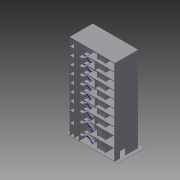
# Autodesk Inventor part: NRCC_Smoke_Tower
Saved by Autodesk Inventor 2013 SP2 (Build 170200200, 200)
## iProperties
Created: 2015-09-15
Part Number: NRCC_Smoke_Tower
Material: Generic
Document SubType Name: Modeling
Designer: mcgratta
Density: 1 g/cm^3
Author: mcgratta
Autodesk Inventor part; units mm, degrees
(part 1 of 2)
sketch "Sketch1" plane through (0, 0, 0) normal (0, 1, 0) x (-1, 0, 0)
  line L0 (-1000, -1000) -> (-1200, -1000)
  line L1 (-1200, -1000) -> (-1200, -10300)
  line L2 (-1200, -10300) -> (-1000, -10300)
  line L3 (-1000, -10300) -> (-1000, -1000)
  line L4 (-1200, -1000) -> (-15700, -1000)
  line L5 (-15700, -1000) -> (-15700, -1200)
  line L6 (-15700, -1200) -> (-1200, -1200)
  line L7 (-1200, -1200) -> (-1200, -1000)
  line L8 (-15700, -1000) -> (-15900, -1000)
  line L9 (-15900, -1000) -> (-15900, -10300)
  line L10 (-15900, -10300) -> (-15700, -10300)
  line L11 (-15700, -10300) -> (-15700, -1000)
  line L12 (-15700, -10300) -> (-15700, -10100)
  line L13 (-1200, -10100) -> (-1200, -10300)
  line L14 (-2400, -2400) -> (-2600, -2400)
  line L15 (-2600, -2400) -> (-2600, -8900)
  line L16 (-2600, -8900) -> (-2400, -8900)
  line L17 (-2400, -8900) -> (-2400, -2400)
  line L18 (-2600, -2400) -> (-11700, -2400)
  line L19 (-11700, -2400) -> (-11700, -2600)
  line L20 (-11700, -2600) -> (-2600, -2600)
  line L21 (-2600, -2600) -> (-2600, -2400)
  line L22 (-2600, -8900) -> (-11700, -8900)
  line L23 (-11700, -8900) -> (-11700, -8700)
  line L24 (-11700, -8700) -> (-2600, -8700)
  line L25 (-2600, -8700) -> (-2600, -8900)
  line L26 (-11700, -8900) -> (-11900, -8900)
  line L27 (-11900, -8900) -> (-11900, -2400)
  line L28 (-11900, -2400) -> (-11700, -2400)
  line L29 (-11700, -2400) -> (-11700, -8900)
  line L30 (-4000, -8700) -> (-4200, -8700)
  line L31 (-4200, -8700) -> (-4200, -2600)
  line L32 (-4200, -2600) -> (-4000, -2600)
  line L33 (-4000, -2600) -> (-4000, -8700)
  line L34 (-2600, -5600) -> (-4000, -5600)
  line L35 (-4000, -5600) -> (-4000, -5400)
  line L36 (-4000, -5400) -> (-2600, -5400)
  line L37 (-2600, -5400) -> (-2600, -5600)
  line L38 (-9200, -8700) -> (-9400, -8700)
  line L39 (-9400, -8700) -> (-9400, -2600)
  line L40 (-9400, -2600) -> (-9200, -2600)
  line L41 (-9200, -2600) -> (-9200, -8700)
  line L42 (-11700, -3900) -> (-11700, -3700)
  line L43 (-9400, -3700) -> (-9400, -3900)
  line L44 (-9400, -5900) -> (-11700, -5900)
  line L45 (-11700, -5900) -> (-11700, -5700)
  line L46 (-11700, -5700) -> (-9400, -5700)
  line L47 (-9400, -5700) -> (-9400, -5900)
  line L48 (-9200, -5900) -> (-9200, -5700)
  line L49 (-4200, -5700) -> (-4200, -5900)
  line L50 (-4200, -5300) -> (-9200, -5300)
  line L51 (-9200, -5300) -> (-9200, -5100)
  line L52 (-9200, -5100) -> (-4200, -5100)
  line L53 (-4200, -5100) -> (-4200, -5300)
  line L54 (-6200, -8700) -> (-6400, -8700)
  line L55 (-6400, -8700) -> (-6400, -5900)
  line L56 (-6400, -5900) -> (-6200, -5900)
  line L57 (-6200, -5900) -> (-6200, -8700)
  line L58 (-7000, -5700) -> (-7200, -5700)
  line L59 (-7200, -5700) -> (-7200, -5300)
  line L60 (-7200, -5300) -> (-7000, -5300)
  line L61 (-7000, -5300) -> (-7000, -5700)
  line L62 (-10200, -5700) -> (-10400, -5700)
  line L63 (-10400, -5700) -> (-10400, -3900)
  line L64 (-10400, -3900) -> (-10200, -3900)
  line L65 (-10200, -3900) -> (-10200, -5700)
  line L66 (-15700, -10300) -> (-1200, -10300)
  line L67 (-1200, -10300) -> (-1200, -10100)
  line L68 (-1200, -10100) -> (-15700, -10100)
  line L69 (-15700, -10100) -> (-15700, -10300)
  line L70 (-11700, -3700) -> (-9400, -3700)
  line L71 (-9400, -3700) -> (-9400, -3900)
  line L72 (-9400, -3900) -> (-11700, -3900)
  line L73 (-11700, -3900) -> (-11700, -3700)
  line L74 (-9200, -5700) -> (-4200, -5700)
  line L75 (-4200, -5700) -> (-4200, -5900)
  line L76 (-4200, -5900) -> (-9200, -5900)
  line L77 (-9200, -5900) -> (-9200, -5700)
  point P0 (0, 0)
  dimension "d0" = 9300
  dimension "d2" = 1000
  dimension "d3" = 1000
  dimension "d4" = 200
  dimension "d5" = 200
  dimension "d6" = 14500
  dimension "d7" = 200
  dimension "d8" = 9300
  dimension "d10" = 1200
  dimension "d11" = 200
  dimension "d12" = 1200
  dimension "d14" = 200
  dimension "d15" = 9100
  dimension "d16" = 200
  dimension "d17" = 9100
  dimension "d18" = 200
  dimension "d19" = 6500
  dimension "d20" = 200
  dimension "d21" = 1400
  dimension "d22" = 200
  dimension "d23" = 2800
  dimension "d24" = 200
  dimension "d25" = 5000
  dimension "d28" = 200
  dimension "d32" = 200
  dimension "d33" = 2500
  dimension "d34" = 200
  dimension "d35" = 2000
  dimension "d36" = 200
  dimension "d37" = 2800
  dimension "d38" = 200
  dimension "d39" = 800
  dimension "d50" = 200
  dimension "d51" = 200
  dimension "d52" = 1200
  dimension "d69" = 200
  dimension "d70" = 1100
  dimension "d71" = 1800
  dimension "d72" = 2800
  dimension "d75" = 400
  dimension "d76" = 2800
  dimension "d77" = 400
  dimension "d78" = 200
  dimension "d79" = 5000
  constraints: 156 end point, 39 parallel, 21 point on line, 18 horizontal, 18 perpendicular
  measures "d0" distance of L0.end L1.end
  measures "d2" distance from line of L0 point (0, 0)
  measures "d3" distance from line of point (0, 0) L3
  measures "d4" distance between parallel lines of L1 L3
  measures "d5" distance between parallel lines of L4 L6
  measures "d6" distance from line of L4.end L1
  measures "d7" distance between parallel lines of L9 L11
  measures "d8" distance from line of L8.end L10
  measures "d10" distance between parallel lines of L17 L1
  measures "d11" distance between parallel lines of L15 L17
  measures "d12" distance between parallel lines of L6 L14
  measures "d14" distance between parallel lines of L18 L20
  measures "d15" distance from line of L19.end L21
  measures "d16" distance between parallel lines of L24 L22
  measures "d17" distance from line of L23 L15.end
  measures "d18" distance between parallel lines of L27 L29
  measures "d19" distance between parallel lines of L26 L28
  measures "d20" distance between parallel lines of L31 L33
  measures "d21" distance between parallel lines of L33 L15
  measures "d22" distance between parallel lines of L36 L34
  measures "d23" distance between parallel lines of L20 L36
  measures "d24" distance between parallel lines of L39 L41
  measures "d25" distance between parallel lines of L41 L31
  measures "d28" distance between parallel lines of L46 L44
  measures "d32" distance between parallel lines of L52 L50
  measures "d33" distance between parallel lines of L20 L52
  measures "d34" distance between parallel lines of L55 L57
  measures "d35" distance between parallel lines of L57 L31
  measures "d36" distance between parallel lines of L59 L61
  measures "d37" distance between parallel lines of L61 L31
  measures "d38" distance between parallel lines of L63 L65
  measures "d39" distance between parallel lines of L65 L39
  measures "d50" distance between parallel lines of L66 L68
  measures "d51" distance between parallel lines of L10 L68
  measures "d52" distance between parallel lines of L68 L22
  measures "d69" distance between parallel lines of L72 L70
  measures "d70" distance between parallel lines of L20 L70
  measures "d71" distance between parallel lines of L46 L64
  measures "d72" distance between parallel lines of L24 L44
  measures "d75" distance between parallel lines of L50 L58
  measures "d76" distance between parallel lines of L24 L56
  measures "d77" distance between parallel lines of L50 L74
  measures "d78" distance between parallel lines of L76 L74
  measures "d79" distance between parallel lines of L77 L75
extrude "Extrusion1" add sketch "Sketch1" along normal blind 27800 contours L3 L2 L1 L0
extrude "Extrusion2" add sketch "Sketch1" along normal blind 27800 contours L5 L11 L10 L9 L8
extrude "Extrusion5" add sketch "Sketch1" along normal blind 27800 contours L1 L6 L5 L4
extrude "Extrusion6" add sketch "Sketch1" along normal blind 27800 contours L66 L11 L68 L1
extrude "Extrusion7" add sketch "Sketch1" along normal blind 27800 contours L15 L20 L19 L18
extrude "Extrusion8" add sketch "Sketch1" along normal blind 27800 contours L17 L16 L15 L14 | L22 L23 L24 L15 | L33 L24 L31 L20 | L24 L55 L56 L57
extrude "Extrusion9" add sketch "Sketch1" along normal blind 27800 contours L15 L34 L33 L36 | L61 L58 L59 L50
extrude "Extrusion10" add sketch "Sketch1" along normal blind 27800 contours L31 L50 L41 L52
extrude "Extrusion11" add sketch "Sketch1" along normal blind 27800 contours L20 L41 L24 L39
extrude "Extrusion12" add sketch "Sketch1" along normal blind 27800 contours L19 L29 L23 L26 L27 L28
extrude "Extrusion13" add sketch "Sketch1" along normal blind 27800 contours L29 L46 L39 L44 | L64 L65 L46 L63
extrude "Extrusion14" add sketch "Sketch1" along normal blind 27800 contours L70 L39 L72 L64 L29
extrude "Extrusion15" add sketch "Sketch1" along normal blind 27800 contours L76 L56 L41 L74 L58 L31
sketch "Sketch3" plane through (1200, 0, -10100) normal (0, 0, 1) x (1, 0, 0)
  line L0 (0, 0) -> (0, 27800) projected
  line L1 (0, 3600) -> (14500, 3600)
  line L2 (14500, 3600) -> (14500, 3400)
  line L3 (14500, 3400) -> (0, 3400)
  line L4 (0, 3400) -> (0, 3600)
  line L5 (0, 7200) -> (14500, 7200)
  line L6 (14500, 7200) -> (14500, 7000)
  line L7 (14500, 7000) -> (0, 7000)
  line L8 (0, 7000) -> (0, 7200)
  line L9 (0, 9800) -> (14500, 9800)
  line L10 (14500, 9800) -> (14500, 9600)
  line L11 (14500, 9600) -> (0, 9600)
  line L12 (0, 9600) -> (0, 9800)
  line L13 (0, 12400) -> (14500, 12400)
  line L14 (14500, 12400) -> (14500, 12200)
  line L15 (14500, 12200) -> (0, 12200)
  line L16 (0, 12200) -> (0, 12400)
  line L17 (0, 15000) -> (14500, 15000)
  line L18 (14500, 15000) -> (14500, 14800)
  line L19 (14500, 14800) -> (0, 14800)
  line L20 (0, 14800) -> (0, 15000)
  line L21 (0, 17600) -> (14500, 17600)
  line L22 (14500, 17600) -> (14500, 17400)
  line L23 (14500, 17400) -> (0, 17400)
  line L24 (0, 17400) -> (0, 17600)
  line L25 (0, 20200) -> (14500, 20200)
  line L26 (14500, 20200) -> (14500, 20000)
  line L27 (14500, 20000) -> (0, 20000)
  line L28 (0, 20000) -> (0, 20200)
  line L29 (0, 22800) -> (14500, 22800)
  line L30 (14500, 22800) -> (14500, 22600)
  line L31 (14500, 22600) -> (0, 22600)
  line L32 (0, 22600) -> (0, 22800)
  line L33 (0, 25400) -> (14500, 25400)
  line L34 (14500, 25400) -> (14500, 25200)
  line L35 (14500, 25200) -> (0, 25200)
  line L36 (0, 25200) -> (0, 25400)
  point P0 (-1200, 0)
  dimension "d97" = 200
  dimension "d99" = 1200
  dimension "d100" = 3400
  dimension "d101" = 14500
  dimension "d102" = 200
  dimension "d103" = 200
  dimension "d104" = 200
  dimension "d105" = 200
  dimension "d106" = 200
  dimension "d107" = 200
  dimension "d108" = 200
  dimension "d109" = 200
  dimension "d110" = 3400
  dimension "d111" = 2400
  dimension "d112" = 2400
  dimension "d113" = 2400
  dimension "d114" = 2400
  dimension "d115" = 2400
  dimension "d116" = 2400
  dimension "d117" = 2400
  dimension "d118" = 1200
  constraints: 72 end point, 18 parallel, 9 horizontal, 9 perpendicular
  measures "d97" distance between parallel lines of L3 L1
  measures "d99" distance from line of point (-1200, 0) L4
  measures "d100" distance from line of point (-1200, 0) L3
  measures "d101" distance between parallel lines of L2 L0
  measures "d102" distance between parallel lines of L7 L5
  measures "d103" distance between parallel lines of L11 L9
  measures "d104" distance between parallel lines of L15 L13
  measures "d105" distance between parallel lines of L19 L17
  measures "d106" distance between parallel lines of L23 L21
  measures "d107" distance between parallel lines of L27 L25
  measures "d108" distance between parallel lines of L31 L29
  measures "d109" distance between parallel lines of L35 L33
  measures "d110" distance between parallel lines of L7 L1
  measures "d111" distance between parallel lines of L11 L5
  measures "d112" distance between parallel lines of L15 L9
  measures "d113" distance between parallel lines of L19 L13
  measures "d114" distance between parallel lines of L17 L23
  measures "d115" distance between parallel lines of L21 L27
  measures "d116" distance between parallel lines of L25 L31
  measures "d117" distance between parallel lines of L29 L35
  measures "d118" distance from line of point (-1200, 0) L0
extrude "Extrusion16" add sketch "Sketch3" along normal blind 8900 contours L0 L1 L2 L3
extrude "Extrusion17" add sketch "Sketch3" along normal blind 8900 contours L0 L33 L34 L35 | L0 L29 L30 L31 | L0 L25 L26 L27 | L0 L21 L22 L23 | L0 L17 L18 L19 | L0 L13 L14 L15 | L0 L9 L10 L11 | L0 L5 L6 L7
sketch "Sketch4" plane through (1200, 25400, -10100) normal (0, 1, 0) x (1, 0, 0)
  line L0 (0, -8900) -> (0, 0) projected
  line L1 (1400, -4700) -> (2800, -4700)
  line L2 (2800, -4700) -> (2800, -7500)
  line L3 (2800, -7500) -> (1400, -7500)
  line L4 (1400, -7500) -> (1400, -4700)
  line L5 (1400, -1400) -> (2800, -1400)
  line L6 (2800, -1400) -> (2800, -4500)
  line L7 (2800, -4500) -> (1400, -4500)
  line L8 (1400, -4500) -> (1400, -1400)
  line L9 (3000, -1400) -> (5000, -1400)
  line L10 (5000, -1400) -> (5000, -4200)
  line L11 (5000, -4200) -> (3000, -4200)
  line L12 (3000, -4200) -> (3000, -1400)
  line L13 (3000, -5000) -> (4500, -5000)
  line L14 (4500, -5000) -> (4500, -7500)
  line L15 (4500, -7500) -> (3000, -7500)
  line L16 (3000, -7500) -> (3000, -5000)
  line L17 (5200, -1400) -> (8000, -1400)
  line L18 (8000, -1400) -> (8000, -4200)
  line L19 (8000, -4200) -> (5200, -4200)
  line L20 (5200, -4200) -> (5200, -1400)
  line L21 (3000, -4400) -> (5800, -4400)
  line L22 (5800, -4400) -> (5800, -4800)
  line L23 (5800, -4800) -> (3000, -4800)
  line L24 (3000, -4800) -> (3000, -4400)
  line L25 (6000, -4400) -> (8000, -4400)
  line L26 (8000, -4400) -> (8000, -4800)
  line L27 (8000, -4800) -> (6000, -4800)
  line L28 (6000, -4800) -> (6000, -4400)
  line L29 (8200, -4400) -> (9000, -4400)
  line L30 (9000, -4400) -> (9000, -6200)
  line L31 (9000, -6200) -> (8200, -6200)
  line L32 (8200, -6200) -> (8200, -4400)
  line L33 (9200, -4400) -> (10500, -4400)
  line L34 (10500, -4400) -> (10500, -6200)
  line L35 (10500, -6200) -> (9200, -6200)
  line L36 (9200, -6200) -> (9200, -4400)
  point P0 (-1200, -10100)
  dimension "d124" = 1400
  dimension "d125" = 1400
  dimension "d126" = 2800
  dimension "d127" = 1400
  dimension "d128" = 200
  dimension "d129" = 1400
  dimension "d130" = 3100
  dimension "d131" = 200
  dimension "d132" = 2000
  dimension "d133" = 2800
  dimension "d134" = 300
  dimension "d135" = 200
  dimension "d137" = 1500
  dimension "d138" = 2500
  dimension "d139" = 200
  dimension "d140" = 2800
  dimension "d141" = 2800
  dimension "d142" = 200
  dimension "d143" = 200
  dimension "d144" = 200
  dimension "d145" = 2800
  dimension "d146" = 200
  dimension "d147" = 200
  dimension "d148" = 400
  dimension "d149" = 2000
  dimension "d150" = 200
  dimension "d151" = 1800
  dimension "d152" = 800
  dimension "d153" = 200
  dimension "d154" = 1300
  dimension "d155" = 1800
  dimension "d156" = 0
  dimension "d159" = 2600
  dimension "d160" = 2600
  constraints: 72 end point, 18 parallel, 9 horizontal, 9 perpendicular, 2 point on line
  measures "d124" distance between parallel lines of L2 L4
  measures "d125" distance between parallel lines of L4 L0
  measures "d126" distance between parallel lines of L3 L1
  measures "d127" distance between parallel lines of L6 L8
  measures "d128" distance between parallel lines of L1 L7
  measures "d129" distance between parallel lines of L0 L8
  measures "d130" distance between parallel lines of L7 L5
  measures "d131" distance between parallel lines of L12 L6
  measures "d132" distance between parallel lines of L10 L12
  measures "d133" distance between parallel lines of L11 L9
  measures "d134" distance between parallel lines of L7 L11
  measures "d135" distance between parallel lines of L16 L2
  measures "d137" distance between parallel lines of L14 L16
  measures "d138" distance between parallel lines of L15 L13
  measures "d139" distance between parallel lines of L20 L10
  measures "d140" distance between parallel lines of L19 L17
  measures "d141" distance between parallel lines of L18 L20
  measures "d142" distance between parallel lines of L21 L11
  measures "d143" distance between parallel lines of L6 L24
  measures "d144" distance between parallel lines of L13 L23
  measures "d145" distance between parallel lines of L22 L24
  measures "d146" distance between parallel lines of L28 L22
  measures "d147" distance between parallel lines of L25 L19
  measures "d148" distance between parallel lines of L27 L25
  measures "d149" distance between parallel lines of L26 L28
  measures "d150" distance between parallel lines of L32 L26
  measures "d151" distance between parallel lines of L31 L29
  measures "d152" distance between parallel lines of L30 L32
  measures "d153" distance between parallel lines of L36 L30
  measures "d154" distance between parallel lines of L34 L36
  measures "d155" distance between parallel lines of L35 L33
  measures "d156" distance between parallel lines of L29 L33
  measures "d159" distance from line of point (-1200, -10100) L15
  measures "d160" distance from line of point (-1200, -10100) L3
extrude "Extrusion18" cut sketch "Sketch4" against normal blind 26000 contours L1 L2 L3 L4 | L5 L6 L7 L8 | L9 L10 L11 L12 | L17 L18 L19 L20 | L21 L22 L23 L24 | L25 L26 L27 L28 | L29 L30 L31 L32 | L33 L34 L35 L36
ref_plane "Work Plane1" through (4200, 27800, -3900) normal (0, 0, 1) x (1, 0, 0)
sketch "Sketch5" plane through (4200, 27800, -3900) normal (0, 0, 1) x (1, 0, 0)
  line L0 (0, -26000) -> (1000, -26000)
  line L1 (1000, -26000) -> (1000, -26050)
  line L2 (1000, -26050) -> (0, -26050)
  line L3 (0, -26050) -> (0, -26000)
  line L4 (3100, -27550) -> (3400, -27550)
  line L5 (3400, -27550) -> (3400, -27600)
  line L6 (3400, -27600) -> (3100, -27600)
  line L7 (3100, -27600) -> (3100, -27550)
  line L8 (2800, -27350) -> (3100, -27350)
  line L9 (3100, -27350) -> (3100, -27400)
  line L10 (3100, -27400) -> (2800, -27400)
  line L11 (2800, -27400) -> (2800, -27350)
  line L12 (2500, -27150) -> (2800, -27150)
  line L13 (2800, -27150) -> (2800, -27200)
  line L14 (2800, -27200) -> (2500, -27200)
  line L15 (2500, -27200) -> (2500, -27150)
  line L16 (2200, -26950) -> (2500, -26950)
  line L17 (2500, -26950) -> (2500, -27000)
  line L18 (2500, -27000) -> (2200, -27000)
  line L19 (2200, -27000) -> (2200, -26950)
  line L20 (1900, -26750) -> (2200, -26750)
  line L21 (2200, -26750) -> (2200, -26800)
  line L22 (2200, -26800) -> (1900, -26800)
  line L23 (1900, -26800) -> (1900, -26750)
  line L24 (1600, -26550) -> (1900, -26550)
  line L25 (1900, -26550) -> (1900, -26600)
  line L26 (1900, -26600) -> (1600, -26600)
  line L27 (1600, -26600) -> (1600, -26550)
  line L28 (1300, -26350) -> (1600, -26350)
  line L29 (1600, -26350) -> (1600, -26400)
  line L30 (1600, -26400) -> (1300, -26400)
  line L31 (1300, -26400) -> (1300, -26350)
  line L32 (1000, -26150) -> (1300, -26150)
  line L33 (1300, -26150) -> (1300, -26200)
  line L34 (1300, -26200) -> (1000, -26200)
  line L35 (1000, -26200) -> (1000, -26150)
  line L36 (0, -22400) -> (1000, -22400)
  line L37 (1000, -22400) -> (1000, -22450)
  line L38 (1000, -22450) -> (0, -22450)
  line L39 (0, -22450) -> (0, -22400)
  line L40 (3100, -23950) -> (3400, -23950)
  line L41 (3400, -23950) -> (3400, -24000)
  line L42 (3400, -24000) -> (3100, -24000)
  line L43 (3100, -24000) -> (3100, -23950)
  line L44 (2800, -23750) -> (3100, -23750)
  line L45 (3100, -23750) -> (3100, -23800)
  line L46 (3100, -23800) -> (2800, -23800)
  line L47 (2800, -23800) -> (2800, -23750)
  line L48 (2500, -23550) -> (2800, -23550)
  line L49 (2800, -23550) -> (2800, -23600)
  line L50 (2800, -23600) -> (2500, -23600)
  line L51 (2500, -23600) -> (2500, -23550)
  line L52 (2200, -23350) -> (2500, -23350)
  line L53 (2500, -23350) -> (2500, -23400)
  line L54 (2500, -23400) -> (2200, -23400)
  line L55 (2200, -23400) -> (2200, -23350)
  line L56 (1900, -23150) -> (2200, -23150)
  line L57 (2200, -23150) -> (2200, -23200)
  line L58 (2200, -23200) -> (1900, -23200)
  line L59 (1900, -23200) -> (1900, -23150)
  line L60 (1600, -22950) -> (1900, -22950)
  line L61 (1900, -22950) -> (1900, -23000)
  line L62 (1900, -23000) -> (1600, -23000)
  line L63 (1600, -23000) -> (1600, -22950)
  line L64 (1300, -22750) -> (1600, -22750)
  line L65 (1600, -22750) -> (1600, -22800)
  line L66 (1600, -22800) -> (1300, -22800)
  line L67 (1300, -22800) -> (1300, -22750)
  line L68 (1000, -22550) -> (1300, -22550)
  line L69 (1300, -22550) -> (1300, -22600)
  line L70 (1300, -22600) -> (1000, -22600)
  line L71 (1000, -22600) -> (1000, -22550)
  line L72 (0, -19400) -> (1100, -19400)
  line L73 (1100, -19400) -> (1100, -19450)
  line L74 (1100, -19450) -> (0, -19450)
  line L75 (0, -19450) -> (0, -19400)
  line L76 (1100, -19600) -> (1400, -19600)
  line L77 (1400, -19600) -> (1400, -19650)
  line L78 (1400, -19650) -> (1100, -19650)
  line L79 (1100, -19650) -> (1100, -19600)
  line L80 (1400, -19800) -> (1700, -19800)
  line L81 (1700, -19800) -> (1700, -19850)
  line L82 (1700, -19850) -> (1400, -19850)
  line L83 (1400, -19850) -> (1400, -19800)
  line L84 (1700, -20000) -> (2000, -20000)
  line L85 (2000, -20000) -> (2000, -20050)
  line L86 (2000, -20050) -> (1700, -20050)
  line L87 (1700, -20050) -> (1700, -20000)
  line L88 (2000, -20200) -> (2300, -20200)
  line L89 (2300, -20200) -> (2300, -20250)
  line L90 (2300, -20250) -> (2000, -20250)
  line L91 (2000, -20250) -> (2000, -20200)
  line L92 (2300, -20400) -> (2600, -20400)
  line L93 (2600, -20400) -> (2600, -20450)
  line L94 (2600, -20450) -> (2300, -20450)
  line L95 (2300, -20450) -> (2300, -20400)
  line L96 (0, -16800) -> (1100, -16800)
  line L97 (1100, -16800) -> (1100, -16850)
  line L98 (1100, -16850) -> (0, -16850)
  line L99 (0, -16850) -> (0, -16800)
  line L100 (1100, -17000) -> (1400, -17000)
  line L101 (1400, -17000) -> (1400, -17050)
  line L102 (1400, -17050) -> (1100, -17050)
  line L103 (1100, -17050) -> (1100, -17000)
  line L104 (1700, -17250) -> (1400, -17250)
  line L105 (1400, -17200) -> (1700, -17200)
  line L106 (1400, -17250) -> (1400, -17200)
  line L107 (1700, -17200) -> (1700, -17250)
  line L108 (2000, -17450) -> (1700, -17450)
  line L109 (1700, -17400) -> (2000, -17400)
  line L110 (1700, -17450) -> (1700, -17400)
  line L111 (2000, -17400) -> (2000, -17450)
  line L112 (2300, -17650) -> (2000, -17650)
  line L113 (2000, -17600) -> (2300, -17600)
  line L114 (2000, -17650) -> (2000, -17600)
  line L115 (2300, -17600) -> (2300, -17650)
  line L116 (2600, -17850) -> (2300, -17850)
  line L117 (2300, -17800) -> (2600, -17800)
  line L118 (2300, -17850) -> (2300, -17800)
  line L119 (2600, -17800) -> (2600, -17850)
  line L120 (0, -14200) -> (1100, -14200)
  line L121 (1100, -14200) -> (1100, -14250)
  line L122 (1100, -14250) -> (0, -14250)
  line L123 (0, -14250) -> (0, -14200)
  line L124 (1100, -14400) -> (1400, -14400)
  line L125 (1400, -14400) -> (1400, -14450)
  line L126 (1400, -14450) -> (1100, -14450)
  line L127 (1100, -14450) -> (1100, -14400)
  line L128 (1700, -14650) -> (1400, -14650)
  line L129 (1400, -14600) -> (1700, -14600)
  line L130 (1400, -14650) -> (1400, -14600)
  line L131 (1700, -14600) -> (1700, -14650)
  line L132 (2000, -14850) -> (1700, -14850)
  line L133 (1700, -14800) -> (2000, -14800)
  line L134 (1700, -14850) -> (1700, -14800)
  line L135 (2000, -14800) -> (2000, -14850)
  line L136 (2300, -15050) -> (2000, -15050)
  line L137 (2000, -15000) -> (2300, -15000)
  line L138 (2000, -15050) -> (2000, -15000)
  line L139 (2300, -15000) -> (2300, -15050)
  line L140 (2600, -15250) -> (2300, -15250)
  line L141 (2300, -15200) -> (2600, -15200)
  line L142 (2300, -15250) -> (2300, -15200)
  line L143 (2600, -15200) -> (2600, -15250)
  line L144 (0, -11600) -> (1100, -11600)
  line L145 (1100, -11600) -> (1100, -11650)
  line L146 (1100, -11650) -> (0, -11650)
  line L147 (0, -11650) -> (0, -11600)
  line L148 (1100, -11800) -> (1400, -11800)
  line L149 (1400, -11800) -> (1400, -11850)
  line L150 (1400, -11850) -> (1100, -11850)
  line L151 (1100, -11850) -> (1100, -11800)
  line L152 (1700, -12050) -> (1400, -12050)
  line L153 (1400, -12000) -> (1700, -12000)
  line L154 (1400, -12050) -> (1400, -12000)
  line L155 (1700, -12000) -> (1700, -12050)
  line L156 (2000, -12250) -> (1700, -12250)
  line L157 (1700, -12200) -> (2000, -12200)
  line L158 (1700, -12250) -> (1700, -12200)
  line L159 (2000, -12200) -> (2000, -12250)
  line L160 (2300, -12450) -> (2000, -12450)
  line L161 (2000, -12400) -> (2300, -12400)
  line L162 (2000, -12450) -> (2000, -12400)
  line L163 (2300, -12400) -> (2300, -12450)
  line L164 (2600, -12650) -> (2300, -12650)
  line L165 (2300, -12600) -> (2600, -12600)
  line L166 (2300, -12650) -> (2300, -12600)
  line L167 (2600, -12600) -> (2600, -12650)
  line L168 (0, -9000) -> (1100, -9000)
  line L169 (1100, -9000) -> (1100, -9050)
  line L170 (1100, -9050) -> (0, -9050)
  line L171 (0, -9050) -> (0, -9000)
  line L172 (1100, -9200) -> (1400, -9200)
  line L173 (1400, -9200) -> (1400, -9250)
  line L174 (1400, -9250) -> (1100, -9250)
  line L175 (1100, -9250) -> (1100, -9200)
  line L176 (1700, -9450) -> (1400, -9450)
  line L177 (1400, -9400) -> (1700, -9400)
  line L178 (1400, -9450) -> (1400, -9400)
  line L179 (1700, -9400) -> (1700, -9450)
  line L180 (2000, -9650) -> (1700, -9650)
  line L181 (1700, -9600) -> (2000, -9600)
  line L182 (1700, -9650) -> (1700, -9600)
  line L183 (2000, -9600) -> (2000, -9650)
  line L184 (2300, -9850) -> (2000, -9850)
  line L185 (2000, -9800) -> (2300, -9800)
  line L186 (2000, -9850) -> (2000, -9800)
  line L187 (2300, -9800) -> (2300, -9850)
  line L188 (2600, -10050) -> (2300, -10050)
  line L189 (2300, -10000) -> (2600, -10000)
  line L190 (2300, -10050) -> (2300, -10000)
  line L191 (2600, -10000) -> (2600, -10050)
  line L192 (0, -6400) -> (1100, -6400)
  line L193 (1100, -6400) -> (1100, -6450)
  line L194 (1100, -6450) -> (0, -6450)
  line L195 (0, -6450) -> (0, -6400)
  line L196 (1100, -6600) -> (1400, -6600)
  line L197 (1400, -6600) -> (1400, -6650)
  line L198 (1400, -6650) -> (1100, -6650)
  line L199 (1100, -6650) -> (1100, -6600)
  line L200 (1700, -6850) -> (1400, -6850)
  line L201 (1400, -6800) -> (1700, -6800)
  line L202 (1400, -6850) -> (1400, -6800)
  line L203 (1700, -6800) -> (1700, -6850)
  line L204 (2000, -7050) -> (1700, -7050)
  line L205 (1700, -7000) -> (2000, -7000)
  line L206 (1700, -7050) -> (1700, -7000)
  line L207 (2000, -7000) -> (2000, -7050)
  line L208 (2300, -7250) -> (2000, -7250)
  line L209 (2000, -7200) -> (2300, -7200)
  line L210 (2000, -7250) -> (2000, -7200)
  line L211 (2300, -7200) -> (2300, -7250)
  line L212 (2600, -7450) -> (2300, -7450)
  line L213 (2300, -7400) -> (2600, -7400)
  line L214 (2300, -7450) -> (2300, -7400)
  line L215 (2600, -7400) -> (2600, -7450)
  line L216 (1400, -4200) -> (1700, -4200)
  line L217 (1700, -4200) -> (1700, -4250)
  line L218 (1700, -4250) -> (1400, -4250)
  line L219 (1700, -4400) -> (2000, -4400)
  line L220 (2000, -4400) -> (2000, -4450)
  line L221 (2000, -4450) -> (1700, -4450)
  line L222 (1700, -4450) -> (1700, -4400)
  line L223 (1400, -4250) -> (1400, -4200)
  line L224 (2000, -4650) -> (2000, -4600)
  line L225 (2300, -4850) -> (2300, -4800)
  line L226 (2300, -4650) -> (2000, -4650)
  line L227 (2300, -4600) -> (2300, -4650)
  line L228 (2600, -4850) -> (2300, -4850)
  line L229 (2600, -4800) -> (2600, -4850)
  line L230 (2300, -4800) -> (2600, -4800)
  line L231 (2000, -4600) -> (2300, -4600)
  line L232 (1100, -3800) -> (1100, -3850)
  line L233 (1100, -4000) -> (1400, -4000)
  line L234 (1400, -4050) -> (1100, -4050)
  line L235 (1100, -4050) -> (1100, -4000)
  line L236 (1100, -3850) -> (0, -3850)
  line L237 (0, -3800) -> (1100, -3800)
  line L238 (0, -3850) -> (0, -3800)
  line L239 (1400, -4000) -> (1400, -4050)
  point P0 (-4200, -27800)
  dimension "d162" = 4200
  dimension "d163" = 5200
  dimension "d164" = 1800
  dimension "d165" = 1750
  dimension "d166" = 50
  dimension "d167" = 300
  dimension "d168" = 200
  dimension "d169" = 7300
  dimension "d170" = 50
  dimension "d171" = 300
  dimension "d172" = 50
  dimension "d173" = 300
  dimension "d174" = 50
  dimension "d175" = 300
  dimension "d176" = 50
  dimension "d177" = 300
  dimension "d178" = 50
  dimension "d179" = 300
  dimension "d180" = 50
  dimension "d181" = 300
  dimension "d182" = 50
  dimension "d183" = 300
  dimension "d184" = 200
  dimension "d185" = 300
  dimension "d186" = 200
  dimension "d187" = 300
  dimension "d188" = 200
  dimension "d189" = 300
  dimension "d190" = 200
  dimension "d191" = 300
  dimension "d192" = 200
  dimension "d193" = 300
  dimension "d194" = 200
  dimension "d195" = 300
  dimension "d196" = 200
  dimension "d197" = 300
  dimension "d198" = 50
  dimension "d199" = 300
  dimension "d200" = 50
  dimension "d201" = 300
  dimension "d202" = 50
  dimension "d203" = 300
  dimension "d204" = 50
  dimension "d205" = 300
  dimension "d206" = 50
  dimension "d207" = 300
  dimension "d208" = 50
  dimension "d209" = 300
  dimension "d210" = 50
  dimension "d211" = 300
  dimension "d212" = 50
  dimension "d213" = 300
  dimension "d214" = 200
  dimension "d215" = 300
  dimension "d216" = 200
  dimension "d217" = 300
  dimension "d218" = 200
  dimension "d219" = 300
  dimension "d220" = 200
  dimension "d221" = 300
  dimension "d222" = 200
  dimension "d223" = 300
  dimension "d224" = 200
  dimension "d225" = 300
  constraints: 480 end point, 120 parallel, 60 horizontal, 60 perpendicular
  measures "d162" distance from line of L3 point (-4200, -27800)
  measures "d163" distance from line of point (-4200, -27800) L1
  measures "d164" distance from line of point (-4200, -27800) L0
  measures "d165" distance from line of point (-4200, -27800) L2
  measures "d166" distance between parallel lines of L6 L4
  measures "d167" distance of L4.end L4.start
  measures "d168" distance from line of point (-4200, -27800) L6
  measures "d169" horizontal distance of point (-4200, -27800) L4.start
  measures "d170" distance between parallel lines of L10 L8
  measures "d171" distance of L8.end L8.start
  measures "d172" distance between parallel lines of L14 L12
  measures "d173" distance of L12.end L12.start
  measures "d174" distance between parallel lines of L18 L16
  measures "d175" distance of L16.end L16.start
  measures "d176" distance between parallel lines of L22 L20
  measures "d177" distance of L20.end L20.start
  measures "d178" distance between parallel lines of L26 L24
  measures "d179" distance of L24.end L24.start
  measures "d180" distance between parallel lines of L30 L28
  measures "d181" distance of L28.end L28.start
  measures "d182" distance between parallel lines of L34 L32
  measures "d183" distance of L32.end L32.start
  measures "d184" distance between parallel lines of L4 L8
  measures "d185" distance between parallel lines of L7 L11
  measures "d186" distance between parallel lines of L8 L12
  measures "d187" distance from line of L11 L12.start
  measures "d188" distance between parallel lines of L16 L12
  measures "d189" distance between parallel lines of L15 L19
  measures "d190" distance between parallel lines of L16 L20
  measures "d191" distance between parallel lines of L19 L23
  measures "d192" distance between parallel lines of L20 L24
  measures "d193" distance between parallel lines of L23 L27
  measures "d194" distance between parallel lines of L24 L28
  measures "d195" distance between parallel lines of L27 L31
  measures "d196" distance between parallel lines of L28 L32
  measures "d197" distance between parallel lines of L31 L35
  measures "d198" distance between parallel lines of L42 L40
  measures "d199" distance of L40.end L40.start
  measures "d200" distance between parallel lines of L46 L44
  measures "d201" distance of L44.end L47.end
  measures "d202" distance between parallel lines of L50 L48
  measures "d203" distance of L48.end L51.end
  measures "d204" distance between parallel lines of L54 L52
  measures "d205" distance of L53.start L55.end
  measures "d206" distance between parallel lines of L58 L56
  measures "d207" distance of L57.start L59.end
  measures "d208" distance between parallel lines of L62 L60
  measures "d209" distance of L61.start L63.end
  measures "d210" distance between parallel lines of L66 L64
  measures "d211" distance of L65.start L64.start
  measures "d212" distance between parallel lines of L70 L68
  measures "d213" distance of L69.start L71.end
  measures "d214" distance between parallel lines of L40 L44
  measures "d215" distance between parallel lines of L43 L47
  measures "d216" distance between parallel lines of L44 L48
  measures "d217" distance from line of L47 L51.end
  measures "d218" distance between parallel lines of L52 L48
  measures "d219" distance between parallel lines of L51 L55
  measures "d220" distance between parallel lines of L52 L56
  measures "d221" distance between parallel lines of L55 L59
  measures "d222" distance between parallel lines of L56 L60
  measures "d223" distance between parallel lines of L59 L63
  measures "d224" distance between parallel lines of L60 L64
  measures "d225" distance between parallel lines of L63 L67
extrude "Extrusion19" add sketch "Sketch5" against normal blind 1200 contours L0 L1 L2 L3 | L4 L5 L6 L7 | L8 L9 L10 L11 | L12 L13 L14 L15 | L16 L17 L18 L19 | L20 L21 L22 L23 | L24 L25 L26 L27 | L28 L29 L30 L31 | L32 L33 L34 L35
extrude "Extrusion20" add sketch "Sketch5" against normal blind 1200 contours L36 L37 L38 L39 | L40 L41 L42 L43 | L44 L45 L46 L47 | L48 L49 L50 L51 | L52 L53 L54 L55 | L56 L57 L58 L59 | L60 L61 L62 L63 | L64 L65 L66 L67 | L68 L69 L70 L71 | L72 L73 L74 L75 | L76 L77 L78 L79 | L80 L81 L82 L83 | L84 L85 L86 L87 | L88 L89 L90 L91 | L92 L93 L94 L95 | L96 L97 L98 L99 | L100 L101 L102 L103 | L104 L106 L105 L107 | L108 L110 L109 L111 | L112 L114 L113 L115 | L116 L118 L117 L119 | L120 L121 L122 L123 | L124 L125 L126 L127 | L128 L130 L129 L131 | L132 L134 L133 L135 | L136 L138 L137 L139 | L140 L142 L141 L143 | L144 L145 L146 L147 | L148 L149 L150 L151 | L152 L154 L153 L155 | L156 L158 L157 L159 | L160 L162 L161 L163 | L164 L166 L165 L167 | L168 L169 L170 L171 | L172 L173 L174 L175 | L176 L178 L177 L179 | L180 L182 L181 L183 | L184 L186 L185 L187 | L188 L190 L189 L191 | L192 L193 L194 L195 | L196 L197 L198 L199 | L200 L202 L201 L203 | L204 L206 L205 L207 | L208 L210 L209 L211 | L212 L214 L213 L215 | L216 L217 L218 L223 | L219 L220 L221 L222 | L224 L231 L227 L226 | L225 L230 L229 L228 | L232 L236 L238 L237 | L233 L239 L234 L235
ref_plane "Work Plane2" through (4200, 27800, -3800) normal (0, 0, 1) x (1, 0, 0)